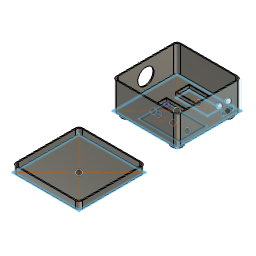
Camera Controller Box v2 (Autodesk Fusion 360 design; units mm, degrees)
Autodesk Fusion 360 part; units mm, degrees
sketch "Sketch1" plane through (0, 0, 0) normal (0, 0, 1) x (1, 0, 0)
  line L0 (0, 0) -> (54.8, 0)
  line L1 (54.8, 0) -> (54.8, -36.6)
  line L2 (54.8, -36.6) -> (0, -36.6)
  line L3 (0, -36.6) -> (0, 0)
  line L4 (-0.1714, 14.8857) -> (43.3286, 14.8857)
  line L5 (43.3286, 14.8857) -> (43.3286, 32.3857)
  line L6 (43.3286, 32.3857) -> (-0.1714, 32.3857)
  line L7 (-0.1714, 32.3857) -> (-0.1714, 14.8857)
  line L8 (44.3295, 13.892) -> (-1.1705, 13.892)
  line L9 (-1.1705, 13.892) -> (-1.1705, 33.392)
  line L10 (-1.1705, 33.392) -> (44.3295, 33.392)
  line L11 (44.3295, 33.392) -> (44.3295, 13.892)
  line L12 (44.3295, 13.892) -> (-1.1705, 33.392) construction
  line L13 (-1.1705, 13.892) -> (44.3295, 33.392) construction
  line L14 (55.8, -37.6) -> (-1, -37.6)
  line L15 (-1, -37.6) -> (-1, 1)
  line L16 (-1, 1) -> (55.8, 1)
  line L17 (55.8, 1) -> (55.8, -37.6)
  line L18 (55.8, -37.6) -> (-1, 1) construction
  line L19 (-1, -37.6) -> (55.8, 1) construction
  line L20 (60, -45) -> (-28, -45)
  line L21 (-28, -45) -> (-28, 43)
  line L22 (-28, 43) -> (60, 43)
  line L23 (60, 43) -> (60, -45)
  line L24 (60, 43) -> (-28, -45) construction
  line L25 (-28, 43) -> (60, -45) construction
  line L26 (61.5, -46.5) -> (-29.5, -46.5)
  line L27 (-29.5, -46.5) -> (-29.5, 44.5)
  line L28 (-29.5, 44.5) -> (61.5, 44.5)
  line L29 (61.5, 44.5) -> (61.5, -46.5)
  line L30 (61.5, -46.5) -> (-29.5, 44.5) construction
  line L31 (-29.5, -46.5) -> (61.5, 44.5) construction
  line L32 (-23.4404, -100.1003) -> (67.5596, -100.1003)
  line L33 (67.5596, -100.1003) -> (67.5596, -191.1003)
  line L34 (67.5596, -191.1003) -> (-23.4404, -191.1003)
  line L35 (-23.4404, -191.1003) -> (-23.4404, -100.1003)
  line L36 (67.5596, -191.1003) -> (-23.4404, -100.1003) construction
  line L37 (-23.4404, -191.1003) -> (67.5596, -100.1003) construction
  line L38 (-24.9404, -98.6003) -> (69.0596, -98.6003)
  line L39 (69.0596, -98.6003) -> (69.0596, -192.6003)
  line L40 (69.0596, -192.6003) -> (-24.9404, -192.6003)
  line L41 (-24.9404, -192.6003) -> (-24.9404, -98.6003)
  line L42 (-24.9404, -98.6003) -> (69.0596, -192.6003) construction
  line L43 (69.0596, -98.6003) -> (-24.9404, -192.6003) construction
  line L44 (6.9, -18.3) -> (47.9, -18.3) construction
  circle A0 centre (47.9, -18.3) radius 1.65
  circle A1 centre (6.9, -18.3) radius 1.65
  line L45 (-1, -15.5) -> (0, -15.5)
  line L46 (0, -15.5) -> (0, -20.5)
  line L47 (0, -20.5) -> (-1, -20.5)
  line L48 (-1, -20.5) -> (-1, -15.5)
  line L49 (-1, -15.5) -> (0, -20.5) construction
  line L50 (0, -15.5) -> (-1, -20.5) construction
  point P0 (21.5795, 23.642)
  point P1 (27.4, -18.3)
  point P2 (16, -1)
  point P3 (22.0596, -145.6003)
  point P4 (22.0596, -145.6003)
  point P5 (-0.5, -18)
  dimension "d1" = 54.8
  dimension "d2" = 36.6
  dimension "d3" = 43.5
  dimension "d4" = 17.5
  dimension "d5" = 45.5
  dimension "d6" = 19.5
  dimension "d7" = 56.8
  dimension "d8" = 38.6
  dimension "d9" = 88
  dimension "d10" = 88
  dimension "d11" = 91
  dimension "d12" = 91
  dimension "d33" = 91
  dimension "d34" = 91
  dimension "d35" = 94
  dimension "d36" = 94
  dimension "d46" = 20.5
  dimension "d47" = 41
  dimension "d48" = 3.3
  dimension "d49" = 3.3
  dimension "d52" = 5
  constraint horizontal L0
  constraint vertical L1
  constraint horizontal L2
  constraint vertical L3
  constraint coincident L0.start L3.end
  constraint horizontal L4
  constraint vertical L5
  constraint horizontal L6
  constraint vertical L7
  constraint horizontal L8
  constraint perpendicular L8 L9
  constraint parallel L8 L10
  constraint parallel L9 L11
  constraint coincident L12 P0
  constraint coincident L13 P0
  constraint horizontal L14
  constraint perpendicular L14 L15
  constraint parallel L14 L16
  constraint parallel L15 L17
  constraint coincident L18 P1
  constraint coincident L19 P1
  constraint horizontal L20
  constraint vertical L21
  constraint horizontal L22
  constraint vertical L23
  constraint horizontal L26
  constraint perpendicular L26 L27
  constraint parallel L26 L28
  constraint parallel L27 L29
  constraint coincident L30 P2
  constraint coincident L31 P2
  constraint midpoint L25 P2
  constraint horizontal L32
  constraint perpendicular L32 L33
  constraint parallel L32 L34
  constraint parallel L33 L35
  constraint horizontal L38
  constraint perpendicular L38 L39
  constraint parallel L38 L40
  constraint parallel L39 L41
  constraint coincident L42 P4
  constraint coincident L43 P4
  constraint coincident P4 P3
  constraint parallel L2 L44
  constraint coincident L44.end A0.centre
  constraint coincident L44.start A1.centre
  constraint horizontal L45
  constraint perpendicular L45 L46
  constraint parallel L45 L47
  constraint parallel L46 L48
  constraint coincident L49 P5
  constraint coincident L50 P5
  measures "d1" distance of L0.start L0.end
  measures "d2" distance of L0.start L2.end
  measures "d3" distance of L4.start L4.end
  measures "d4" distance of L4.start L6.end
  measures "d5" distance of L9.end L10.end
  measures "d6" distance of L8.end L9.end
  measures "d7" distance of L15.end L16.end
  measures "d8" distance of L14.end L15.end
  measures "d9" distance of L20.start L20.end
  measures "d10" distance of L20.start L22.end
  measures "d11" distance of L27.end L28.end
  measures "d12" distance of L26.end L27.end
  measures "d33" distance of L33.end L34.end
  measures "d34" distance of L32.end L33.end
  measures "d35" distance of L39.end L40.end
  measures "d36" distance of L38.end L39.end
  measures "d46" distance of P1 L44.start
  measures "d47" distance of L44.start L44.end
  measures "d48" diameter of A0
  measures "d49" diameter of A1
  measures "d52" distance of L45.end L46.end
extrude "Extrude1" add sketch "Sketch1" along normal blind 40 contours L26 L27 L28 L29 makes body 1
extrude "Extrude2" add sketch "Sketch1" along normal blind 3 contours L20 L21 L22 L23 bodies 1
extrude "Extrude3" add sketch "Sketch1" along normal blind 7 contours L0 L1 L2 L3 L14 L15 L16 L17 L45 L47 | L8 L9 L10 L11 bodies 1
extrude "Extrude4" add sketch "Sketch1" along normal blind 3 contours L0 L1 L2 L3 L46 | L4 L5 L6 L7 | A0 | A1 bodies 1
sketch "Sketch2" plane through (-29.5, 0, 0) normal (-1, 0, 0) x (0, -1, 0)
  line L0 (-44.5, 0) -> (46.5, 0)
  line L1 (46.5, 0) -> (46.5, 40)
  line L2 (46.5, 40) -> (-44.5, 40)
  line L3 (-44.5, 40) -> (-44.5, 0)
  line L4 (-44.5, 40) -> (46.5, 0) construction
  line L5 (46.5, 40) -> (-44.5, 0) construction
  circle A0 centre (1, 20) radius 11.5
  dimension "d21" = 23
  constraint coincident L2.end L3.start
  constraint coincident L0.end L1.start
  constraint coincident L1.end L2.start
  constraint coincident L0.start L3.end
  constraint midpoint L4 A0.centre
  measures "d21" diameter of A0
extrude "Extrude5" cut sketch "Sketch2" against normal up to surface (1.5 mm away) contours A0 bodies 1
sketch "Sketch3" plane through (61.5, 0, 0) normal (1, 0, 0) x (0, 1, 0)
  line L0 (-46.5, 0) -> (44.5, 0)
  line L1 (44.5, 0) -> (44.5, 40)
  line L2 (44.5, 40) -> (-46.5, 40)
  line L3 (-46.5, 40) -> (-46.5, 0)
  line L4 (32, 7.35) -> (18, 7.35)
  line L5 (18, 7.35) -> (18, 12.65)
  line L6 (18, 12.65) -> (32, 12.65)
  line L7 (32, 12.65) -> (32, 7.35)
  line L8 (32, 7.35) -> (18, 12.65) construction
  line L9 (18, 7.35) -> (32, 12.65) construction
  circle A0 centre (25, 22) radius 2.95
  circle A1 centre (12.4967, 22) radius 2.5
  point P0 (25, 10)
  dimension "d24" = 14
  dimension "d25" = 5.3
  dimension "d28" = 5.9
  dimension "d43" = 5
  constraint horizontal L4
  constraint perpendicular L4 L5
  constraint parallel L4 L6
  constraint parallel L5 L7
  constraint coincident L8 P0
  constraint coincident L9 P0
  measures "d24" distance of L5.end L6.end
  measures "d25" distance of L4.end L5.end
  measures "d28" diameter of A0
  measures "d43" diameter of A1
extrude "Extrude6" cut sketch "Sketch3" against normal up to surface (1.5 mm away) contours L4 L5 L6 L7 bodies 1
extrude "Extrude7" cut sketch "Sketch3" against normal up to surface (1.5 mm away) contours A0 bodies 1
fillet "Fillet1" radius 5 8 edges at (61.5, 44.5, 20) (60, 43, 21.5) (-28, 43, 21.5) (-29.5, 44.5, 20) (-28, -45, 21.5) (-29.5, -46.5, 20) (61.5, -46.5, 20) (60, -45, 21.5) on bodies 1
extrude "Extrude8" add sketch "Sketch1" along normal blind 2 separate body contours L32 L33 L34 L35 makes body 2
extrude "Extrude9" add sketch "Sketch1" along normal blind 10 contours L38 L39 L40 L41 bodies 2
fillet "Fillet2" radius 5 8 edges at (-23.4404, -191.1003, 6) (-24.9404, -98.6003, 5) (-23.4404, -100.1003, 6) (-24.9404, -192.6003, 5) (67.5596, -191.1003, 6) (69.0596, -192.6003, 5) (69.0596, -98.6003, 5) (67.5596, -100.1003, 6) on bodies 2
extrude "Extrude10" cut sketch "Sketch3" against normal up to surface (1.5 mm away) contours A1 bodies 1
extrude "Extrude11" add sketch "Sketch1" along normal blind 8 contours A0 | A1 bodies 1
extrude "Extrude12" add sketch "Sketch1" along normal up to surface (3 mm away) contours L3 L15 L45 L46 L47 L48 bodies 1
sketch "Sketch4" plane through (0, 0, 0) normal (0, 0, 1) x (1, 0, 0)
  line L0 (3.5, -13.5) -> (28.5, -13.5)
  line L1 (28.5, -13.5) -> (28.5, 11.5)
  line L2 (28.5, 11.5) -> (3.5, 11.5)
  line L3 (3.5, 11.5) -> (3.5, -13.5)
  line L4 (3.5, -13.5) -> (28.5, 11.5) construction
  line L5 (28.5, -13.5) -> (3.5, 11.5) construction
  line L6 (16, -1) -> (-19.3553, 34.3553) construction
  line L7 (16, -1) -> (51.3553, 34.3553) construction
  line L8 (16, -1) -> (-19.3553, -36.3553) construction
  line L9 (16, -1) -> (51.3553, -36.3553) construction
  circle A0 centre (-19.3553, 34.3553) radius 7.5
  circle A1 centre (51.3553, 34.3553) radius 7.5
  circle A2 centre (-19.3553, -36.3553) radius 7.5
  circle A3 centre (51.3553, -36.3553) radius 7.5
  point P0 (16, -1)
  dimension "d55" = 25
  dimension "d56" = 25
  dimension "d57" = 50
  dimension "d58" = 50
  dimension "d59" = 50
  dimension "d60" = 50
  dimension "d61" = 15
  dimension "d62" = 15
  dimension "d63" = 15
  dimension "d64" = 15
  constraint horizontal L0
  constraint perpendicular L0 L1
  constraint parallel L0 L2
  constraint parallel L1 L3
  constraint coincident L4 P0
  constraint coincident L5 P0
  constraint coincident P0 L6.start
  constraint perpendicular L4 L6
  constraint perpendicular L6 L7
  constraint perpendicular L6 L8
  constraint parallel L5 L9
  constraint coincident L6.end A0.centre
  constraint coincident L7.end A1.centre
  constraint coincident L8.end A2.centre
  constraint coincident L9.end A3.centre
  measures "d55" distance of L1.end L2.end
  measures "d56" distance of L0.end L1.end
  measures "d57" distance of P0 L6.end
  measures "d58" distance of P0 L7.end
  measures "d59" distance of P0 L8.end
  measures "d60" distance of P0 L9.end
  measures "d61" diameter of A0
  measures "d62" diameter of A1
  measures "d63" diameter of A2
  measures "d64" diameter of A3
extrude "Extrude13" add sketch "Sketch4" against normal blind 5 bodies 1
hole "Hole1" at (16, -1, -5) direction (0, 0, 1) diameter 5.118 depth 4.8 tip angle 118 bodies 1
thread "Thread1" "ANSI Unified Screw Threads 0.25 1/4-20 UNC 1B" thread offset 0 thread depth 7.4
fillet "Fillet3" radius 8.5 4 edges at (28.5, 11.5, -2.5) (3.5, 11.5, -2.5) (3.5, -13.5, -2.5) (28.5, -13.5, -2.5) on bodies 1
equation "d5 = d3 + 2 mm"
equation "d6 = d4 + 2 mm"
equation "d7 = d1 + 2 mm"
equation "d8 = d2 + 2 mm"
equation "d11 = d10 + 3 mm"
equation "d12 = d9 + 3 mm"
equation "d33 = d12"
equation "d35 = d33 + 3 mm"
equation "d36 = d34 + 3 mm"
